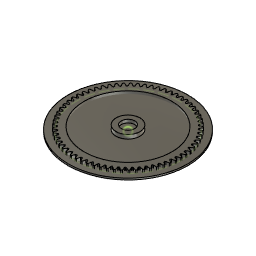
Turntable v1 (Autodesk Fusion 360 design; units mm, degrees)
description: Spur Gear; Module: 2.0; Num Teeth: 65; Pressure Angle: 20.0; Backlash: 0.15 mm
Autodesk Fusion 360 part; units mm, degrees
sketch "Sketch1" plane through (0, 0, 0) normal (0, 0, 1) x (1, 0, 0)
  circle A0 centre (0, 0) radius 75
  dimension "d1" = 150
  constraint coincident A0.centre origin
  measures "d1" diameter of A0
extrude "Extrude1" add sketch "Sketch1" along normal blind 2 makes body 1
sketch "Sketch2" plane through (0, 0, 2) normal (0, 0, 1) x (-1, 0, 0)
  circle A0 centre (0, 0) radius 75
  circle A1 centre (0, 0) radius 65
  dimension "d4" = 130
  constraint coincident A0.centre A1.centre
  measures "d4" diameter of A1
sketch "Sketch1 (2)" plane through (0, 0, 0) normal (0, 0, 1) x (1, 0, 0) in component "Spur Gear (65 teeth)"
  circle A0 centre (0, 0) radius 62.5492
  circle A1 centre (0, 0) radius 55
extrude "Extrude1'" add sketch "Sketch1 (2)" along normal blind 5 separate body makes body 2 in component "Spur Gear (65 teeth)"
sketch "Sketch2 (2)" plane through (0, 0, 0) normal (0, 0, 1) x (1, 0, 0) in component "Spur Gear (65 teeth)"
  spline S0 degree 5 poles (61.0348, -2.3506) (61.052, -2.3506) (61.0865, -2.3503) (61.1381, -2.3496) (61.2071, -2.3478) (61.2932, -2.3443) (61.3794, -2.3394) (61.4655, -2.3334) (61.5516, -2.3261) (61.6378, -2.3177) (61.7239, -2.3084) (61.81, -2.2982) (61.8961, -2.2872) (61.9822, -2.2755) (62.0683, -2.2632) (62.1543, -2.2502) (62.2403, -2.2367) (62.3263, -2.2225) (62.4122, -2.2076) (62.4982, -2.1922) (62.5841, -2.1761) (62.6699, -2.1595) (62.7558, -2.1424) (62.8416, -2.1247) (62.9274, -2.1065) (63.0131, -2.0878) (63.0988, -2.0687) (63.1845, -2.049) (63.2701, -2.0289) (63.3557, -2.0082) (63.4413, -1.9872) (63.5268, -1.9656) (63.6123, -1.9436) (63.6978, -1.9212) (63.7832, -1.8983) (63.8686, -1.875) (63.954, -1.8513) (64.0393, -1.8272) (64.1245, -1.8027) (64.2097, -1.7777) (64.2949, -1.7524) (64.3801, -1.7266) (64.4651, -1.7005) (64.5502, -1.674) (64.6352, -1.647) (64.7202, -1.6198) (64.8051, -1.5921) (64.89, -1.5641) (64.9748, -1.5357) (65.0596, -1.5069) (65.1443, -1.4778) (65.229, -1.4483) (65.3136, -1.4184) (65.3982, -1.3882) (65.4828, -1.3577) (65.5673, -1.3268) (65.6517, -1.2955) (65.7361, -1.264) (65.8205, -1.2321) (65.9047, -1.1998) (65.989, -1.1672) (66.0732, -1.1343) (66.1573, -1.1011) (66.2414, -1.0675) (66.3255, -1.0336) (66.4094, -0.9994) (66.4934, -0.9649) (66.5772, -0.93) (66.6611, -0.8949) (66.7448, -0.8594) (66.8285, -0.8236) (66.8955, -0.7947) (66.9456, -0.7729) (66.9791, -0.7583) (66.9958, -0.751) knots 0 0 0 0 0 0 0.01428571 0.02857143 0.04285714 0.05714286 0.07142857 0.08571429 0.1 0.11428571 0.12857143 0.14285714 0.15714286 0.17142857 0.18571429 0.2 0.21428571 0.22857143 0.24285714 0.25714286 0.27142857 0.28571429 0.3 0.31428571 0.32857143 0.34285714 0.35714286 0.37142857 0.38571429 0.4 0.41428571 0.42857143 0.44285714 0.45714286 0.47142857 0.48571429 0.5 0.51428571 0.52857143 0.54285714 0.55714286 0.57142857 0.58571429 0.6 0.61428571 0.62857143 0.64285714 0.65714286 0.67142857 0.68571429 0.7 0.71428571 0.72857143 0.74285714 0.75714286 0.77142857 0.78571429 0.8 0.81428571 0.82857143 0.84285714 0.85714286 0.87142857 0.88571429 0.9 0.91428571 0.92857143 0.94285714 0.95714286 0.97142857 0.98571429 1 1 1 1 1 1
  spline S1 degree 5 poles (61.0348, 2.3506) (61.052, 2.3506) (61.0865, 2.3503) (61.1381, 2.3496) (61.2071, 2.3478) (61.2932, 2.3443) (61.3794, 2.3394) (61.4655, 2.3334) (61.5516, 2.3261) (61.6378, 2.3177) (61.7239, 2.3084) (61.81, 2.2982) (61.8961, 2.2872) (61.9822, 2.2755) (62.0683, 2.2632) (62.1543, 2.2502) (62.2403, 2.2367) (62.3263, 2.2225) (62.4122, 2.2076) (62.4982, 2.1922) (62.5841, 2.1761) (62.6699, 2.1595) (62.7558, 2.1424) (62.8416, 2.1247) (62.9274, 2.1065) (63.0131, 2.0878) (63.0988, 2.0687) (63.1845, 2.049) (63.2701, 2.0289) (63.3557, 2.0082) (63.4413, 1.9872) (63.5268, 1.9656) (63.6123, 1.9436) (63.6978, 1.9212) (63.7832, 1.8983) (63.8686, 1.875) (63.954, 1.8513) (64.0393, 1.8272) (64.1245, 1.8027) (64.2097, 1.7777) (64.2949, 1.7524) (64.3801, 1.7266) (64.4651, 1.7005) (64.5502, 1.674) (64.6352, 1.647) (64.7202, 1.6198) (64.8051, 1.5921) (64.89, 1.5641) (64.9748, 1.5357) (65.0596, 1.5069) (65.1443, 1.4778) (65.229, 1.4483) (65.3136, 1.4184) (65.3982, 1.3882) (65.4828, 1.3577) (65.5673, 1.3268) (65.6517, 1.2955) (65.7361, 1.264) (65.8205, 1.2321) (65.9047, 1.1998) (65.989, 1.1672) (66.0732, 1.1343) (66.1573, 1.1011) (66.2414, 1.0675) (66.3255, 1.0336) (66.4094, 0.9994) (66.4934, 0.9649) (66.5772, 0.93) (66.6611, 0.8949) (66.7448, 0.8594) (66.8285, 0.8236) (66.8955, 0.7947) (66.9456, 0.7729) (66.9791, 0.7583) (66.9958, 0.751) knots 0 0 0 0 0 0 0.01428571 0.02857143 0.04285714 0.05714286 0.07142857 0.08571429 0.1 0.11428571 0.12857143 0.14285714 0.15714286 0.17142857 0.18571429 0.2 0.21428571 0.22857143 0.24285714 0.25714286 0.27142857 0.28571429 0.3 0.31428571 0.32857143 0.34285714 0.35714286 0.37142857 0.38571429 0.4 0.41428571 0.42857143 0.44285714 0.45714286 0.47142857 0.48571429 0.5 0.51428571 0.52857143 0.54285714 0.55714286 0.57142857 0.58571429 0.6 0.61428571 0.62857143 0.64285714 0.65714286 0.67142857 0.68571429 0.7 0.71428571 0.72857143 0.74285714 0.75714286 0.77142857 0.78571429 0.8 0.81428571 0.82857143 0.84285714 0.85714286 0.87142857 0.88571429 0.9 0.91428571 0.92857143 0.94285714 0.95714286 0.97142857 0.98571429 1 1 1 1 1 1
  arc A0 (66.9958, -0.751) -> (66.9958, 0.751) centre (0, 0) ccw
  line L0 (61.0348, 2.3506) -> (61.0348, -2.3506)
  point P0 (61.4586, -2.3336)
  point P1 (61.8834, -2.2887)
  point P2 (62.3089, -2.2252)
  point P3 (62.7347, -2.1465)
  point P4 (63.1609, -2.0543)
  point P5 (63.5873, -1.95)
  point P6 (64.0137, -1.8344)
  point P7 (64.4402, -1.7081)
  point P8 (64.8667, -1.5717)
  point P9 (65.293, -1.4256)
  point P10 (65.7192, -1.2702)
  point P11 (66.145, -1.1059)
  point P12 (66.5706, -0.9327)
  point P13 (61.4586, 2.3336)
  point P14 (61.8834, 2.2887)
  point P15 (62.3089, 2.2252)
  point P16 (62.7347, 2.1465)
  point P17 (63.1609, 2.0543)
  point P18 (63.5873, 1.95)
  point P19 (64.0137, 1.8344)
  point P20 (64.4402, 1.7081)
  point P21 (64.8667, 1.5717)
  point P22 (65.293, 1.4256)
  point P23 (65.7192, 1.2702)
  point P24 (66.145, 1.1059)
  point P25 (66.5706, 0.9327)
extrude "Extrude2" add sketch "Sketch2 (2)" along normal blind 5 bodies 2 in component "Spur Gear (65 teeth)"
fillet "Fillet1" radius 1 2 edges at (62.5109, 2.1897, 2.5) (62.5109, -2.1897, 2.5) on bodies 2 in component "Spur Gear (65 teeth)"
pattern_circular "C-Pattern1" count 65 over 360 about axis through (0, 0, 0) along (0, 0, 1) of "Extrude2", "Fillet1" in component "Spur Gear (65 teeth)"
sketch "Sketch3" plane through (0, 0, 0) normal (0, 0, 1) x (1, 0, 0) in component "Spur Gear (65 teeth)"
  circle A0 centre (0, 0) radius 65 construction
sketch "Sketch3 (2)" plane through (0, 0, 2) normal (0, 0, 1) x (-1, 0, 0)
  circle A0 centre (0, 0) radius 15
  dimension "d13" = 30
  constraint coincident A0.centre origin
  measures "d13" diameter of A0
extrude "Extrude2'" add sketch "Sketch3 (2)" along normal blind 5 bodies 1
hole "Hole3" at (0, 0, 7) direction (0, 0, -1) diameter 16.95 depth 4 tip angle 180 bodies 1
hole "Hole2" [suppressed]
hole "Hole1" [suppressed]
extrude "Extrude3" [suppressed]
extrude "Extrude4" [suppressed]
component "Spur Gear (65 teeth)" placed x (1, 0, 0) y (0, 1, 0) z (0, 0, 1) at (0, 0, 0)
equation "distanceOne = 5.00 mm"
equation "taperAngle1 = 0.0 deg"
equation "Radius = 1.00 mm"
equation "countU = 65"
